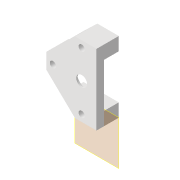
# Autodesk Inventor part: Assembly_Cube_Z_Focus_MGN_NEMA_belt_pushing_cage_v3
Saved by Autodesk Inventor 2022 (Build 260153000, 153)
## iProperties
Created: 2021-12-20
Part Number: Assembly_Cube_Z_Focus_MGN_NEMA_belt_pushing_cage_v3
Material: Generisch
Document SubType Name: Modeling
Designer: diederichbenedict
Density: 1 g/cm^3
Appearance: Vorgabe
Author: diederichbenedict
Autodesk Inventor part; units mm, degrees
ref_plane "YZ Plane" through (0, 0, 0) normal (1, 0, 0) x (0, 1, 0)
ref_plane "XZ Plane" through (0, 0, 0) normal (0, 1, 0) x (-1, 0, 0)
ref_plane "Arbeitsebene1" through (0, 0, 1) normal (0, 0, 1) x (1, 0, 0)
sketch "Skizze1" plane through (0, 0, 1) normal (0, 0, 1) x (1, 0, 0)
  circle A0 centre (-16.4298, 19.2591) radius 1.4 projected
  circle A1 centre (-3.4298, 6.2591) radius 1.4 projected
  circle A2 centre (-3.4298, 32.2591) radius 1.4 projected
  circle A3 centre (-3.43, 19.2591) radius 2.45 construction
  line L0 (-0.43, 35.2591) -> (-6.43, 35.2591)
  line L1 (-6.43, 35.2591) -> (-6.43, 3.2591)
  line L2 (-6.43, 3.2591) -> (-0.43, 3.2591)
  line L3 (-0.43, 3.2591) -> (-0.43, 35.2591)
  line L4 (-0.43, 35.2591) -> (-6.43, 3.2591) construction
  line L5 (-6.43, 35.2591) -> (-0.43, 3.2591) construction
  line L6 (-6.43, 22.7591) -> (-19.43, 22.7591)
  line L7 (-19.43, 22.7591) -> (-19.43, 15.7591)
  line L8 (-19.43, 15.7591) -> (-6.43, 15.7591)
  line L9 (-6.43, 15.7591) -> (-6.43, 22.7591)
  line L10 (-6.43, 22.7591) -> (-19.43, 15.7591) construction
  line L11 (-19.43, 22.7591) -> (-6.43, 15.7591) construction
  line L12 (-6.43, 3.2591) -> (-19.43, 15.7591)
  line L13 (-19.43, 22.7591) -> (-6.43, 35.2591)
  line L14 (-0.43, 3.2591) -> (3.27, 3.2591)
  line L15 (3.27, 3.2591) -> (3.27, 35.2591)
  line L16 (3.27, 35.2591) -> (-0.43, 35.2591)
  line L17 (-0.43, 35.2591) -> (-0.43, 3.2591)
  circle A4 centre (-3.43, 19.2591) radius 1.5
  point P0 (0, 0)
  point P1 (-12.93, 19.2591)
  point P2 (-6.43, 19.2591)
  dimension "d1" = 6
  dimension "d2" = 32
  dimension "d3" = 7
  dimension "d4" = 13
  dimension "d12" = 3.7
  dimension "d18" = 3
  constraints: 36 end point, 6 midpoint, 6 parallel, 3 horizontal, 3 perpendicular, 1 centre point, 1 coincident
  measures "d1" distance of L2.end L1.end
  measures "d2" distance of L1.end L0.end
  measures "d3" distance of L7.end L6.end
  measures "d4" distance between parallel lines of L9 L7
  measures "d12" distance of L16.end L15.end
  measures "d18" diameter of A4
extrude "Extrusion1" add sketch "Skizze1" along normal blind 3.4
sketch "Skizze2" plane through (0, 0, 1) normal (0, 0, -1) x (-1, 0, 0)
  circle A0 centre (3.4298, 32.2591) radius 1.4 projected
  line L0 (16.86, 34.56) -> (16.86, 4.56) projected
  circle A1 centre (16.4298, 19.2591) radius 1.4 projected
  circle A2 centre (3.4298, 6.2591) radius 1.4 projected
  line L1 (6.43, 35.2591) -> (19.43, 22.7591) projected
  line L2 (19.43, 22.7591) -> (19.43, 15.7591) projected
  line L3 (19.43, 15.7591) -> (6.43, 3.2591) projected
  circle A3 centre (16.4298, 19.2591) radius 1.4 projected
  circle A4 centre (3.4298, 6.2591) radius 1.4 projected
  circle A5 centre (3.4298, 32.2591) radius 1.4 projected
  line L4 (-3.27, 29.2591) -> (12.67, 29.2591)
  line L5 (6.43, 35.2591) -> (19.43, 22.7591) projected
  line L6 (19.43, 22.7591) -> (19.43, 15.7591) projected
  line L7 (19.43, 22.7591) -> (13.43, 22.7591)
  line L8 (13.43, 22.7591) -> (13.43, 15.7591)
  line L9 (13.43, 15.7591) -> (19.43, 15.7591)
  line L10 (-3.27, 9.2591) -> (12.67, 9.2591)
  line L11 (19.43, 15.7591) -> (6.43, 3.2591) projected
  line L12 (6.43, 3.2591) -> (-3.27, 3.2591) projected
  line L13 (-3.27, 3.2591) -> (-3.27, 35.2591) projected
  line L14 (-3.27, 35.2591) -> (6.43, 35.2591) projected
  point P0 (0, 0)
  point P1 (12.67, 29.2591)
  dimension "d8" = 6
  dimension "d13" = 6
  dimension "d14" = 6
  constraints: 10 end point, 4 point on line, 3 horizontal, 3 perpendicular
  measures "d8" distance between parallel lines of L8 L2
  measures "d13" distance between parallel lines of L4 L14
  measures "d14" distance between parallel lines of L12 L10
extrude "Extrusion2" add sketch "Skizze2" along normal blind 6.7 contours L7 L2 L9 L0 A1 | L0 A1 L9 L8 L7 | L4 L13 L14 L1 | L10 L3 L12 L13
sketch "Skizze4" plane through (0, 0, 1) normal (0, 0, -1) x (-1, 0, 0)
  circle A0 centre (3.43, 19.2591) radius 1.5 projected
  circle A1 centre (3.43, 19.2591) radius 4
  point P0 (0, 0)
  dimension "d19" = 8
  constraints: 1 centre point, 1 coincident
  measures "d19" diameter of A1
extrude "Extrusion4" cut sketch "Skizze4" against normal blind 3
